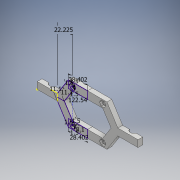
# Autodesk Inventor part: Mousetrap holders
Saved by Autodesk Inventor 2018 (Build 220112000, 112)
## iProperties
Created: 2018-02-06
Part Number: Mousetrap holders
Material: Generic
Document SubType Name: Modeling
Designer: Payal Jindal
Density: 1 g/cm^3
Appearance: Default
Author: Payal Jindal
Autodesk Inventor part; units mm, degrees
ref_plane "YZ Plane" through (0, 0, 0) normal (1, 0, 0) x (0, 1, 0)
ref_plane "XZ Plane" through (0, 0, 0) normal (0, 1, 0) x (-1, 0, 0)
ref_plane "XY Plane" through (0, 0, 0) normal (0, 0, 1) x (1, 0, 0)
sketch "Sketch1" plane through (0, 0, 0) normal (0, 0, 1) x (1, 0, 0)
  line L0 (0, 0) -> (0, 7)
  line L1 (0, 7) -> (10, 7)
  arc A0 (10, 7) -> (19.5394, 7) centre (14.7697, 8.5) ccw
  line L2 (19.5394, 7) -> (29.5394, 7)
  line L3 (29.5394, 7) -> (29.5394, 0)
  line L4 (29.5394, 0) -> (0, 0)
  dimension "d0" = 1.5
  dimension "d1" = 10
  dimension "d2" = 7
  dimension "d3" = 5
  constraints: 10 end point, 3 perpendicular, 2 collinear, 2 point on circle, 1 centre point, 1 horizontal
  measures "d0" distance from line of L1 A0.centre
  measures "d1" distance of L0.end L1.end
  measures "d2" distance of L0.start L0.end
  measures "d3" radius of A0
extrude "Extrusion1" add sketch "Sketch1" along normal blind 10
sketch "Sketch2" plane through (0, 0, 0) normal (0, -1, 0) x (1, 0, 0)
  line L0 (51.7644, 5) -> (51.7644, 29.7066) construction
  line L1 (51.7644, 5) -> (51.7644, -19.6) construction
  line L2 (29.5394, 0) -> (29.5394, 10) projected
  line L3 (29.5394, 10) -> (19.5394, 10) projected
  line L4 (47.1317, 29.7066) -> (49.448, 33.7186)
  line L5 (49.448, 33.7186) -> (54.0808, 33.7186)
  line L6 (54.0808, 33.7186) -> (56.3971, 29.7066)
  line L7 (56.3971, 29.7066) -> (54.0808, 25.6945)
  line L8 (54.0808, 25.6945) -> (49.448, 25.6945)
  line L9 (49.448, 25.6945) -> (47.1317, 29.7066)
  line L10 (49.4261, -15.55) -> (54.1027, -15.55)
  line L11 (54.1027, -15.55) -> (56.4409, -19.6)
  line L12 (56.4409, -19.6) -> (54.1027, -23.65)
  line L13 (54.1027, -23.65) -> (49.4261, -23.65)
  line L14 (49.4261, -23.65) -> (47.0879, -19.6)
  line L15 (47.0879, -19.6) -> (49.4261, -15.55)
  line L16 (74.0252, 24.1945) -> (45.6317, 24.1945)
  line L17 (45.6317, 35.2186) -> (74.0332, 35.2186)
  line L18 (73.9894, -25.15) -> (45.5879, -25.15)
  line L19 (73.9974, -14.05) -> (45.5879, -14.05)
  line L20 (45.5879, -25.15) -> (45.5879, -14.05)
  line L21 (45.6317, 35.2186) -> (45.6317, 24.1945)
  line L22 (45.5879, -25.15) -> (29.5394, 0)
  line L23 (29.5394, 10) -> (45.6317, 35.2186)
  line L24 (29.5394, 5) -> (39.5162, 5)
  line L25 (39.5162, 5) -> (51.6722, -14.05)
  line L26 (39.5162, 5) -> (51.7644, 24.1945)
  line L27 (74.0332, 35.2186) -> (74.0252, 24.1945)
  line L28 (73.9894, -25.15) -> (73.9974, -14.05)
  point P0 (0, 0)
  dimension "d12" = 22.225
  dimension "d22" = 1.5
  dimension "d23" = 1.5
  dimension "d25" = 11.1
  dimension "d29" = 11.1
  dimension "d30" = 28.4015
  dimension "d31" = 28.4015
  dimension "d32" = 122.542
  dimension "d33" = 8.1
  dimension "d34" = 1.5
  dimension "d35" = 1.5
  dimension "d36" = 1.5
  dimension "d37" = 1.5
  constraints: 54 end point, 7 horizontal, 4 vertical, 3 point on line, 2 coincident, 2 parallel, 1 collinear, 1 midpoint, 26 other
  measures "d12" distance between parallel lines of L0 L2
  measures "d22" distance from line of L20 L14.end
  measures "d23" distance from line of L4.start L21
  measures "d25" distance between parallel lines of L22 L25
  measures "d29" distance between parallel lines of L26 L23
  measures "d30" distance of L17.start L17.end
  measures "d31" distance of L18.start L18.end
  measures "d32" angle of L16 L26
  measures "d33" distance between parallel lines of L13 L10
  measures "d34" distance between parallel lines of L17 L5
  measures "d35" distance between parallel lines of L16 L8
  measures "d36" distance between parallel lines of L19 L10
  measures "d37" distance between parallel lines of L18 L13
extrude "Extrusion2" add sketch "Sketch2" against normal blind 7 contours L2 L24 L25 L19 L20 L22 | L2 L23 L21 L16 L26 L24 | L20 L19 L28 L18 | L17 L27 L16 L21 | L4 L5 L6 L7 L8 L9 | L10 L11 L12 L13 L14 L15
extrude "Extrusion3" cut sketch "Sketch2" against normal blind 3.125 contours L4 L5 L6 L7 L8 L9 | L10 L11 L12 L13 L14 L15
hole "Hole1" at (51.7644, 0, 29.7066) at (51.7644, 0, -19.6) direction (0, 1, 0) diameter 4.305 end through all clearance for "Flat Head Machine Screw (82)" size "#6" standard "Ansi Unified Screw Threads"
mirror "Mirror1" about plane through (74.0332, 0, 35.2186) normal (0.9999997, 0, -0.0007255) of "Extrusion2", "Extrusion1", "Extrusion3", "Hole1"
body "Solid1"
